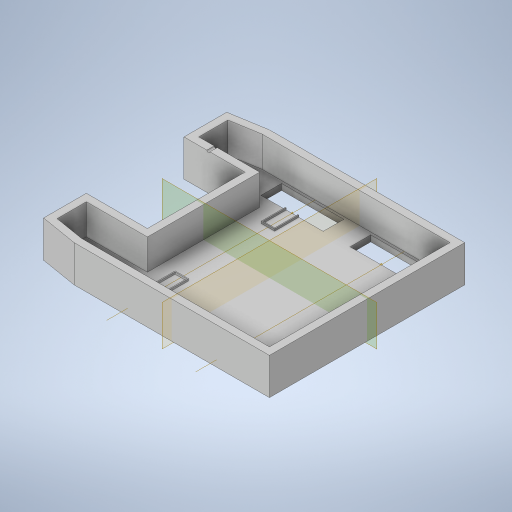
# Autodesk Inventor part: Bot v1 bottom
Saved by Autodesk Inventor 2024 (Build 280153000, 153)
## iProperties
Created: 2023-09-24
Part Number: Bot v1 bottom
Material: Generic
Document SubType Name: Modeling
Designer: CJ110
Density: 1 g/cm^3
Appearance: Default
Author: CJ110
Autodesk Inventor part; units mm, degrees
ref_plane "YZ Plane" through (0, 0, 0) normal (1, 0, 0) x (0, 1, 0)
ref_plane "XZ Plane" through (0, 0, 0) normal (0, 1, 0) x (-1, 0, 0)
ref_plane "XY Plane" through (0, 0, 0) normal (0, 0, 1) x (1, 0, 0)
sketch "Sketch1" plane through (0, 0, 0) normal (0, 1, 0) x (-1, 0, 0)
  line L0 (0, 0) -> (203.2, 0)
  line L1 (203.2, 0) -> (203.2, 203.2)
  line L2 (203.2, 203.2) -> (0, 203.2)
  line L3 (0, 203.2) -> (0, 0)
  dimension "Body_Length" = 203.2
  dimension "Body_Width" = 203.2
  constraints: 8 end point, 2 parallel, 1 horizontal, 1 perpendicular
  measures "Body_Length" distance of L0.start L0.end
  measures "Body_Width" distance of L2.end L0.start
extrude "Base" add sketch "Sketch1" along normal blind 6.35
sketch "Sketch3" plane through (0, 6.35, 0) normal (0, 1, 0) x (1, 0, 0)
  line L0 (-203.2, 0) -> (-203.2, -203.2) projected
  line L1 (-203.2, -203.2) -> (0, -203.2) projected
  line L2 (0, -203.2) -> (0, 0) projected
  line L3 (0, 0) -> (-203.2, 0) projected
  line L4 (-195.58, -7.62) -> (-7.62, -7.62)
  line L5 (-7.62, -7.62) -> (-7.62, -195.58)
  line L6 (-7.62, -195.58) -> (-195.58, -195.58)
  line L7 (-195.58, -195.58) -> (-195.58, -160.02)
  line L8 (-177.8, -152.4) -> (-177.8, -50.8)
  line L9 (-195.58, -43.18) -> (-195.58, -7.62)
  line L10 (-203.2, 0) -> (-203.2, -203.2) projected
  line L11 (-195.58, -160.02) -> (-170.18, -160.02)
  line L12 (-170.18, -160.02) -> (-170.18, -43.18)
  line L13 (-170.18, -43.18) -> (-195.58, -43.18)
  line L14 (-177.8, -152.4) -> (-203.2, -152.4)
  line L15 (-177.8, -50.8) -> (-203.2, -50.8)
  dimension "Wall_Thickness" = 7.62
  dimension "Cuttout_Width" = 101.6
  dimension "Cuttout_Depth" = 25.4
  dimension "d30" = 7.62
  dimension "d31" = 7.62
  dimension "d32" = 7.62
  dimension "d33" = 7.62
  constraints: 22 end point, 5 perpendicular, 3 point on line, 2 vertical, 1 collinear, 2 other
  measures "Wall_Thickness" distance between parallel lines of L1 L6
  measures "Cuttout_Width" distance of L8.start L8.end
  measures "Cuttout_Depth" distance between parallel lines of L0 L8
  measures "d30" distance between parallel lines of L0 L7
  measures "d31" distance between parallel lines of L11 L14
  measures "d32" distance between parallel lines of L13 L15
  measures "d33" distance between parallel lines of L8 L12
extrude "Wall" add sketch "Sketch3" along normal blind 31.75 contours L3 L2 L1 L0 L14 L8 L15
sketch "Sketch7" plane through (0, 6.35, 0) normal (0, 1, 0) x (1, 0, 0)
  line L0 (-203.2, -50.8) -> (-203.2, -152.4) projected
  line L1 (-203.2, -152.4) -> (-177.8, -152.4) projected
  line L2 (-177.8, -152.4) -> (-177.8, -50.8) projected
  line L3 (-177.8, -50.8) -> (-203.2, -50.8) projected
  point P0 (0, 0)
extrude "Cuttout" cut sketch "Sketch7" against normal through all
sketch "Sketch2" plane through (0, 6.35, 0) normal (0, 1, 0) x (1, 0, 0)
  line L0 (-180.34, -193.04) -> (-115.57, -193.04)
  line L1 (-115.57, -193.04) -> (-115.57, -171.45)
  line L2 (-115.57, -171.45) -> (-180.34, -171.45)
  line L3 (-180.34, -171.45) -> (-180.34, -193.04)
  line L4 (-87.63, -193.04) -> (-22.86, -193.04)
  line L5 (-22.86, -193.04) -> (-22.86, -171.45)
  line L6 (-22.86, -171.45) -> (-87.63, -171.45)
  line L7 (-87.63, -171.45) -> (-87.63, -193.04)
  line L8 (-203.2, 0) -> (-203.2, -203.2) projected
  line L9 (-203.2, -203.2) -> (0, -203.2) projected
  line L10 (0, -203.2) -> (0, 0) projected
  line L11 (-203.2, -101.6) -> (0, -101.6) construction
  line L12 (-180.34, -10.16) -> (-115.57, -10.16)
  line L13 (-115.57, -10.16) -> (-115.57, -31.75)
  line L14 (-115.57, -31.75) -> (-180.34, -31.75)
  line L15 (-180.34, -31.75) -> (-180.34, -10.16)
  line L16 (-87.63, -10.16) -> (-22.86, -10.16)
  line L17 (-22.86, -10.16) -> (-22.86, -31.75)
  line L18 (-22.86, -31.75) -> (-87.63, -31.75)
  line L19 (-87.63, -31.75) -> (-87.63, -10.16)
  line L20 (-101.6, -203.2) -> (-101.6, 0) construction
  line L21 (0, 0) -> (-203.2, 0) projected
  line L22 (-7.62, -195.58) -> (-195.58, -195.58) projected
  line L23 (-195.58, -195.58) -> (-195.58, -160.02) projected
  point P0 (-22.86, -182.245)
  point P1 (-22.86, -20.955)
  dimension "Wheel_Hole_Width" = 21.59
  dimension "Wheel_Hole_Diameter" = 64.77
  dimension "d8" = 64.77
  dimension "d11" = 21.59
  dimension "Wheel_Distance_Side" = 2.54
  dimension "d21" = 13.97
  dimension "d22" = 13.97
  dimension "Wheel_Distance_Front" = 15.24
  constraints: 36 end point, 9 symmetric about line, 5 midpoint, 4 parallel, 2 horizontal, 2 perpendicular, 1 collinear
  measures "Wheel_Hole_Width" distance between parallel lines of L0 L2
  measures "Wheel_Hole_Diameter" distance of L0.start L0.end
  measures "d8" distance of L4.start L4.end
  measures "d11" distance between parallel lines of L4 L6
  measures "Wheel_Distance_Side" distance between parallel lines of L22 L0
  measures "d21" distance between parallel lines of L20 L1
  measures "d22" distance between parallel lines of L20 L7
  measures "Wheel_Distance_Front" distance between parallel lines of L23 L3
extrude "Wheels" cut sketch "Sketch2" against normal up to next contours L3 L2 L1 L0 | L7 L6 L5 L4 | L12 L13 L14 L15 | L16 L17 L18 L19
ref_plane "Work Plane2" through (0, 0, 101.6) normal (0, 0, -1) x (-1, 0, 0)
ref_plane "Work Plane3" through (-101.6, 0, 203.2) normal (1, 0, 0) x (0, 0, -1)
sketch "Sketch11" plane through (0, 38.1, 0) normal (0, 1, 0) x (1, 0, 0)
  line L0 (-195.58, -43.18) -> (-195.58, -7.62) projected
  line L1 (-203.2, 0) -> (-203.2, -203.2) projected
  line L2 (-195.58, -7.62) -> (-203.2, -7.62)
  line L3 (-203.2, -7.62) -> (-203.2, -43.18)
  line L4 (-203.2, -43.18) -> (-195.58, -43.18)
  line L5 (-195.58, -43.18) -> (-195.58, -7.62)
  line L6 (-170.18, -160.02) -> (-195.58, -160.02) projected
  line L7 (-203.2, -152.4) -> (-203.2, -203.2) projected
  line L8 (-195.58, -160.02) -> (-203.2, -160.02)
  line L9 (-203.2, -160.02) -> (-203.2, -195.58)
  line L10 (-203.2, -195.58) -> (-195.58, -195.58)
  line L11 (-195.58, -195.58) -> (-195.58, -160.02)
  line L12 (-170.18, -43.18) -> (-195.58, -43.18) projected
  line L13 (-7.62, -195.58) -> (-195.58, -195.58) projected
  point P0 (0, 0)
  point P1 (-203.2, -50.8)
  constraints: 16 end point, 4 parallel, 2 collinear, 2 horizontal, 2 perpendicular, 2 point on line
extrude "Extrusion11" cut sketch "Sketch11" against normal up to surface (31.75 mm away)
sketch "Sketch12" plane through (0, 0, 0) normal (0, -1, 0) x (1, 0, 0)
  line L0 (-180.34, 31.75) -> (-115.57, 31.75) projected
  line L1 (-115.57, 31.75) -> (-115.57, 10.16) projected
  line L2 (-115.57, 10.16) -> (-180.34, 10.16) projected
  line L3 (-180.34, 10.16) -> (-180.34, 31.75) projected
  line L4 (-22.86, 171.45) -> (-87.63, 171.45) projected
  line L5 (-87.63, 171.45) -> (-87.63, 193.04) projected
  line L6 (-87.63, 193.04) -> (-22.86, 193.04) projected
  line L7 (-22.86, 193.04) -> (-22.86, 171.45) projected
  line L8 (-22.86, 31.75) -> (-22.86, 10.16) projected
  line L9 (-22.86, 10.16) -> (-87.63, 10.16) projected
  line L10 (-87.63, 10.16) -> (-87.63, 31.75) projected
  line L11 (-87.63, 31.75) -> (-22.86, 31.75) projected
  line L12 (-115.57, 171.45) -> (-180.34, 171.45) projected
  line L13 (-180.34, 171.45) -> (-180.34, 193.04) projected
  line L14 (-180.34, 193.04) -> (-115.57, 193.04) projected
  line L15 (-115.57, 193.04) -> (-115.57, 171.45) projected
  line L16 (-177.8, 50.8) -> (-203.2, 50.8) projected
  line L17 (-203.2, 0) -> (-203.2, 50.8) projected
  line L18 (0, 0) -> (-203.2, 0) projected
  line L19 (0, 203.2) -> (0, 0) projected
  line L20 (-203.2, 203.2) -> (0, 203.2) projected
  line L21 (-203.2, 152.4) -> (-203.2, 203.2) projected
  line L22 (-203.2, 152.4) -> (-177.8, 152.4) projected
  line L23 (-177.8, 152.4) -> (-177.8, 50.8) projected
  line L24 (-7.62, 195.58) -> (-203.2, 195.58) projected
  line L25 (-203.2, 195.58) -> (-203.2, 203.2) projected
  line L26 (-203.2, 203.2) -> (0, 203.2) projected
  line L27 (0, 203.2) -> (0, 0) projected
  line L28 (0, 0) -> (-203.2, 0) projected
  line L29 (-203.2, 0) -> (-203.2, 7.62) projected
  line L30 (-203.2, 7.62) -> (-7.62, 7.62) projected
  line L31 (-7.62, 7.62) -> (-7.62, 195.58) projected
  line L32 (-203.2, 160.02) -> (-170.18, 160.02) projected
  line L33 (-170.18, 160.02) -> (-170.18, 43.18) projected
  line L34 (-170.18, 43.18) -> (-203.2, 43.18) projected
  line L35 (-203.2, 43.18) -> (-203.2, 50.8) projected
  line L36 (-203.2, 50.8) -> (-177.8, 50.8) projected
  line L37 (-177.8, 50.8) -> (-177.8, 152.4) projected
  line L38 (-177.8, 152.4) -> (-203.2, 152.4) projected
  line L39 (-203.2, 152.4) -> (-203.2, 160.02) projected
  line L40 (-203.2, 0) -> (-241.3, 6.35)
  line L41 (-241.3, 6.35) -> (-241.3, 50.8)
  line L42 (-241.3, 50.8) -> (-203.2, 50.8)
  line L43 (-203.2, 7.62) -> (-233.68, 12.7)
  line L44 (-233.68, 12.7) -> (-233.68, 43.18)
  line L45 (-233.68, 43.18) -> (-203.2, 43.18)
  line L46 (-177.8, 50.8) -> (-177.8, 152.4) projected
  line L47 (-177.8, 101.6) -> (0, 101.6) construction
  line L48 (-203.2, 203.2) -> (-241.3, 196.85)
  line L49 (-241.3, 196.85) -> (-241.3, 152.4)
  line L50 (-241.3, 152.4) -> (-203.2, 152.4)
  line L51 (-203.2, 195.58) -> (-233.68, 190.5)
  line L52 (-233.68, 190.5) -> (-233.68, 160.02)
  line L53 (-233.68, 160.02) -> (-203.2, 160.02)
  dimension "d52" = 7.62
  dimension "d53" = 38.1
  dimension "d54" = 44.45
  constraints: 26 end point, 6 symmetric about line, 2 horizontal, 2 midpoint, 2 parallel, 1 vertical
  measures "d52" distance between parallel lines of L41 L44
  measures "d53" distance between parallel lines of L17 L41
  measures "d54" distance of L40.end L41.end
extrude "Extrusion12" add sketch "Sketch12" against normal up to surface (6.35 mm away) contours L17 L45 L44 L43 L40 L41 L42 | L17 L43 L44 L45 | L50 L49 L48 L21 L51 L52 L53 | L53 L52 L51 L21
extrude "Extrusion13" add sketch "Sketch12" against normal up to surface (38.1 mm away) contours L17 L45 L44 L43 L40 L41 L42 | L50 L49 L48 L21 L51 L52 L53
sketch "Sketch13" plane through (-177.8, 0, 50.8) normal (0, 0, 1) x (1, 0, 0)
  line L0 (0, 0) -> (-63.5, 0) projected
  line L1 (0, 38.1) -> (0, 0) projected
  line L2 (0, 38.1) -> (-63.5, 38.1) projected
  line L3 (-63.5, 0) -> (-63.5, 38.1) projected
  line L4 (-63.5, 38.1) -> (0, 38.1) projected
  circle A0 centre (-38.1, 38.1) radius 1.55
  point P0 (177.8, 0)
  point P1 (-39.65, 38.1)
  point P2 (-36.55, 38.1)
  point P3 (-31.75, 38.1)
  dimension "d59" = 3.1
  dimension "d62" = 31.75
  constraints: 1 centre point, 1 midpoint, 1 point on line
  measures "d59" diameter of A0
  measures "d62" distance of L1.start point (-31.75, 38.1)
extrude "Extrusion14" cut sketch "Sketch13" against normal up to surface (7.62 mm away) contours A0 L2 picked at (-37.7623, 37.311)
sketch "Sketch14" plane through (0, 6.35, 0) normal (0, 1, 0) x (1, 0, 0)
  line L0 (-180.34, -171.45) -> (-115.57, -171.45) projected
  line L1 (-153.98, -171.45) -> (-141.93, -171.45)
  line L2 (-141.93, -171.45) -> (-141.93, -147.4)
  line L3 (-141.93, -147.4) -> (-153.98, -147.4)
  line L4 (-153.98, -147.4) -> (-153.98, -171.45)
  line L5 (-147.955, -243.84) -> (-147.955, 40.64) construction
  line L6 (-154.98, -171.45) -> (-140.93, -171.45)
  line L7 (-140.93, -171.45) -> (-140.93, -146.4)
  line L8 (-140.93, -146.4) -> (-154.98, -146.4)
  line L9 (-154.98, -146.4) -> (-154.98, -171.45)
  line L10 (-170.18, -43.18) -> (-170.18, -160.02) projected
  line L11 (-170.18, -101.6) -> (-7.62, -101.6) construction
  line L12 (-7.62, -195.58) -> (-7.62, -7.62) projected
  line L13 (-141.93, -31.75) -> (-141.93, -55.8)
  line L14 (-141.93, -55.8) -> (-153.98, -55.8)
  line L15 (-153.98, -55.8) -> (-153.98, -31.75)
  line L16 (-147.955, 40.64) -> (-147.955, -243.84) construction
  line L17 (-140.93, -31.75) -> (-140.93, -56.8)
  line L18 (-140.93, -56.8) -> (-154.98, -56.8)
  line L19 (-154.98, -56.8) -> (-154.98, -31.75)
  line L20 (-233.68, -190.5) -> (-203.2, -195.58) projected
  line L21 (-203.2, -195.58) -> (-7.62, -195.58) projected
  line L22 (-7.62, -195.58) -> (-7.62, -7.62) projected
  line L23 (-203.2, -7.62) -> (-7.62, -7.62) projected
  line L24 (-203.2, -7.62) -> (-233.68, -12.7) projected
  line L25 (-233.68, -12.7) -> (-233.68, -43.18) projected
  line L26 (-233.68, -43.18) -> (-170.18, -43.18) projected
  line L27 (-170.18, -43.18) -> (-170.18, -160.02) projected
  line L28 (-170.18, -160.02) -> (-233.68, -160.02) projected
  line L29 (-233.68, -160.02) -> (-233.68, -190.5) projected
  line L30 (-115.57, -31.75) -> (-180.34, -31.75) projected
  line L31 (-180.34, -31.75) -> (-180.34, -10.16) projected
  line L32 (-180.34, -10.16) -> (-115.57, -10.16) projected
  line L33 (-115.57, -10.16) -> (-115.57, -31.75) projected
  line L34 (-87.63, -171.45) -> (-22.86, -171.45) projected
  line L35 (-22.86, -171.45) -> (-22.86, -193.04) projected
  line L36 (-22.86, -193.04) -> (-87.63, -193.04) projected
  line L37 (-87.63, -193.04) -> (-87.63, -171.45) projected
  line L38 (-22.86, -10.16) -> (-22.86, -31.75) projected
  line L39 (-22.86, -31.75) -> (-87.63, -31.75) projected
  line L40 (-87.63, -31.75) -> (-87.63, -10.16) projected
  line L41 (-87.63, -10.16) -> (-22.86, -10.16) projected
  line L42 (-180.34, -171.45) -> (-115.57, -171.45) projected
  line L43 (-115.57, -171.45) -> (-115.57, -193.04) projected
  line L44 (-115.57, -193.04) -> (-180.34, -193.04) projected
  line L45 (-180.34, -193.04) -> (-180.34, -171.45) projected
  point P0 (0, 0)
  dimension "d64" = 12.05
  dimension "d65" = 6.025
  dimension "d66" = 24.05
  dimension "d67" = 1
  dimension "d68" = 1
  dimension "d69" = 1
  constraints: 32 end point, 10 symmetric about line, 4 parallel, 2 horizontal, 2 midpoint, 2 perpendicular, 2 point on line
  measures "d64" distance between parallel lines of L2 L4
  measures "d65" distance between parallel lines of L4 L5
  measures "d66" distance of L3.end L1.start
  measures "d67" distance between parallel lines of L3 L8
  measures "d68" distance between parallel lines of L2 L7
  measures "d69" distance between parallel lines of L4 L9
extrude "Extrusion15" add sketch "Sketch14" along normal blind 2 contours L9 L8 L7 L0 L2 L3 L4 | L30 L17 L18 L19 L15 L14 L13
equation "\"d30\" = Wall_Thickness"
equation "\"d31\" = Wall_Thickness"
equation "\"d32\" = Wall_Thickness"
equation "\"d33\" = Wall_Thickness"
equation "\"d8\" = Wheel_Hole_Diameter"
equation "\"d11\" = Wheel_Hole_Width"
equation "\"d22\" = d21"
equation "\"d52\" = Wall_Thickness"
equation "\"d65\" = 0.5 * d64"
equation "\"d68\" = d67"
equation "\"d69\" = d68"
body "Solid1"
